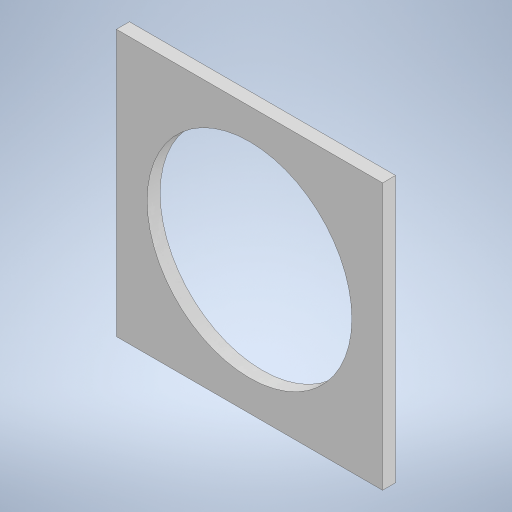
# Autodesk Inventor part: square with hole
Saved by Autodesk Inventor 2023 (Build 270158000, 158)
## iProperties
Created: 2023-02-28
Part Number: square with hole
Material: Generic
Document SubType Name: Modeling
Designer: torba
Density: 1 g/cm^3
Appearance: Default
Author: torba
Autodesk Inventor part; units mm, degrees
ref_plane "YZ Plane" through (0, 0, 0) normal (1, 0, 0) x (0, 1, 0)
ref_plane "XZ Plane" through (0, 0, 0) normal (0, 1, 0) x (-1, 0, 0)
ref_plane "XY Plane" through (0, 0, 0) normal (0, 0, 1) x (1, 0, 0)
sketch "Sketch1" plane through (0, 0, 0) normal (0, 0, 1) x (1, 0, 0)
  circle A0 centre (0, 0) radius 25
  line L0 (-32.5, -32.5) -> (32.5, -32.5)
  line L1 (32.5, -32.5) -> (32.5, 32.5)
  line L2 (32.5, 32.5) -> (-32.5, 32.5)
  line L3 (-32.5, 32.5) -> (-32.5, -32.5)
  line L4 (-32.5, -32.5) -> (32.5, 32.5) construction
  line L5 (32.5, -32.5) -> (-32.5, 32.5) construction
  dimension "d0" = 50
  dimension "d1" = 65
  dimension "d2" = 65
  constraints: 12 end point, 2 midpoint, 2 parallel, 1 centre point, 1 coincident, 1 horizontal, 1 perpendicular
  measures "d0" diameter of A0
  measures "d1" distance of L2.end L1.end
  measures "d2" distance of L1.end L0.end
extrude "Extrusion1" add sketch "Sketch1" along normal blind 3.175
body "Solid1"
